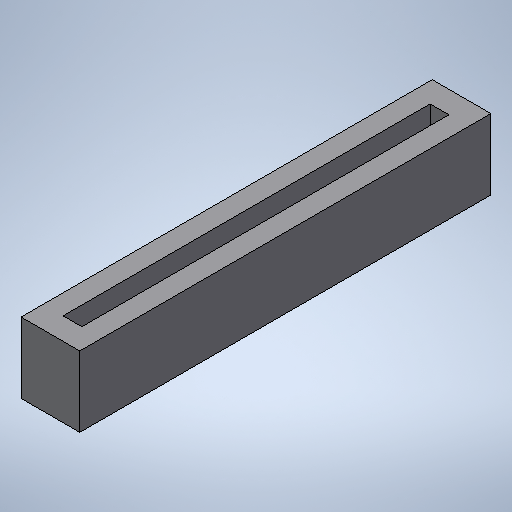
# Autodesk Inventor part: riser7pin
Saved by Autodesk Inventor 2025.3 (Build 293356000, 356)
## iProperties
Created: 2026-01-14
Part Number: riser7pin
Project: COMMON
Material: Generic
Catalog Web Link: https://www.janelia.org/
Vendor: HHMI: JRC - JET
Document SubType Name: Modeling
Designer: sawtelles
Density: 1 g/cm^3
Appearance: Default
RuleStatus: InUse
AfterDocSave0: file://Part Number Cleaner
Title: Standard
Author: sawtelles
Revision Number: 0
LAB/DEPT: COMMON
REQUESTING SCIENTIST: COMMON
DESIGN DEPARTMENT: HHMI: JRC - ID&F
ALTERED ITEM PART NUMBER: N/A
ALTERED ITEM VENDOR: N/A
ALTERED ITEM DESCRIPTION: N/A
Autodesk Inventor part; units mm, degrees
ref_plane "YZ Plane" through (0, 0, 0) normal (1, 0, 0) x (0, 1, 0)
ref_plane "XZ Plane" through (0, 0, 0) normal (0, 1, 0) x (-1, 0, 0)
ref_plane "XY Plane" through (0, 0, 0) normal (0, 0, 1) x (1, 0, 0)
sketch "Sketch1" plane through (0, 0, 0) normal (0, 1, 0) x (-1, 0, 0)
  line L0 (-1.27, -8.89) -> (1.27, -8.89)
  line L1 (1.27, -8.89) -> (1.27, 8.89)
  line L2 (1.27, 8.89) -> (-1.27, 8.89)
  line L3 (-1.27, 8.89) -> (-1.27, -8.89)
  line L4 (-1.27, -8.89) -> (1.27, 8.89) construction
  line L5 (1.27, -8.89) -> (-1.27, 8.89) construction
  line L6 (-0.4064, -7.9375) -> (0.4064, -7.9375)
  line L7 (0.4064, -7.9375) -> (0.4064, 7.9375)
  line L8 (0.4064, 7.9375) -> (-0.4064, 7.9375)
  line L9 (-0.4064, 7.9375) -> (-0.4064, -7.9375)
  line L10 (-0.4064, -7.9375) -> (0.4064, 7.9375) construction
  line L11 (0.4064, -7.9375) -> (-0.4064, 7.9375) construction
  point P0 (0, 0)
  dimension "d0" = 2.54
  dimension "d1" = 17.78
  dimension "d2" = 0.8128
  dimension "d3" = 15.875
  constraints: 24 end point, 4 midpoint, 4 parallel, 2 horizontal, 2 perpendicular
  measures "d0" distance of L2.end L1.end
  measures "d1" distance of L1.end L0.end
  measures "d2" distance of L8.end L7.end
  measures "d3" distance of L7.end L6.end
extrude "Extrusion1" add sketch "Sketch1" along normal blind 3.048
body "Solid1"
